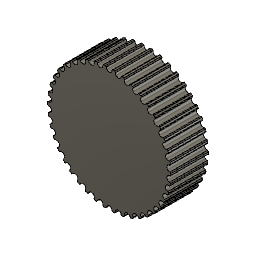
HTD 5M - Universal v3 v3 (Autodesk Fusion 360 design; units mm, degrees)
Autodesk Fusion 360 part; units mm, degrees
sketch "Sketch1" plane through (0, 0, 0) normal (0, 0, 1) x (1, 0, 0) in component "HTD 5M Pulley"
  circle A0 centre (0, 0) radius 32.851
  line L0 (0, 0) -> (0, 32.316) construction
  arc A1 (-1.5246, 32.3519) -> (-1.9804, 32.7913) centre (-1.9545, 32.3621) ccw
  arc A2 (-1.5246, 32.3519) -> (1.5246, 32.3519) centre (0, 32.316) ccw
  arc A3 (1.9804, 32.7913) -> (1.5246, 32.3519) centre (1.9545, 32.3621) ccw
  dimension "d12" = 3.05
  dimension "d19" = 65.7021
  dimension "d20" = 30.791
  dimension "d21" = 0.43
  constraint coincident A0.centre L0.start
  constraint coincident L0.end A2.centre
  constraint tangent A1 A2
  constraint tangent A0 A1
  constraint coincident A0 A1.end
  constraint vertical L0
  constraint tangent A0 A3
  constraint tangent A2 A3
  constraint coincident A0 A3.start
  constraint equal A1 A3
  measures "d12" diameter of A2
  measures "d19" diameter of A0
  measures "d20" distance of A0.centre A2
  measures "d21" radius of A1
extrude "Extrude1" add sketch "Sketch1" along normal blind 20 in component "HTD 5M Pulley"
extrude "Extrude2" cut sketch "Sketch1" along normal blind 20 contours A0 A1 A2 A3 picked at (0, 32.1599) in component "HTD 5M Pulley"
pattern_circular "C-Pattern1" count 42 over 360 about axis through (0, 0, 1.75) along (0, 0, 1) of "Extrude2" in component "HTD 5M Pulley"
component "HTD 5M Pulley" placed x (1, 0, 0) y (0, 1, 0) z (0, 0, 1) at (0, 0, 0)
equation "Teeth = 42" comment "Enter number of teeth"
equation "Pitch = 5 mm"
equation "OutsideDia = 2 * ( ( Teeth * Pitch ) / ( PI * 2 ) - PitchLineOffset )"
equation "PitchLineOffset = 0.5715 mm"
equation "ToothDia = 2.06 mm"
equation "MinorDia = OutsideDia - 2 * ToothDia"
equation "ToothWidth = 3.05 mm"
equation "ToothRootDia = 0.86 mm"
equation "d12 = ToothWidth"
equation "d17 = 20 mm"
equation "d19 = OutsideDia"
equation "d20 = MinorDia / 2"
equation "d21 = ToothRootDia / 2"
equation "d22 = d17"
equation "d24 = Teeth"
